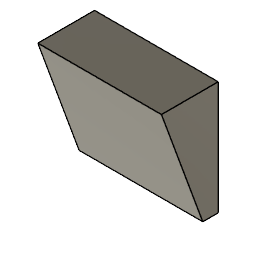
Front Mount (Autodesk Fusion 360 archive; units mm, degrees)
design "Front Bracket"
part number: 2026-01-01-12-06-02-870
Autodesk Fusion 360 part; units mm, degrees
sketch "Sketch1" plane through (0, 0, 0) normal (0, 1, 0) x (1, 0, 0)
  line L0 (0, 0) -> (38, 0)
  line L1 (38, 0) -> (38, -38)
  line L2 (38, -38) -> (0, -38)
  line L3 (0, -38) -> (0, 0)
  circle A0 centre (5, -5) radius 1.35
  circle A1 centre (33, -5) radius 1.35
  circle A2 centre (5, -33) radius 1.35
  circle A3 centre (33, -33) radius 1.35
  line L4 (5, -5) -> (0, -5)
  dimension "d1" = 38
  dimension "d2" = 38
  dimension "d3" = 2.7
  dimension "d4" = 5
  dimension "d5" = 5
  dimension "d6" = 2.7
  dimension "d7" = 2.7
  dimension "d8" = 2.7
  dimension "d9" = 5
  dimension "d10" = 5
  dimension "d11" = 5
  dimension "d12" = 5
  dimension "d13" = 5
  dimension "d14" = 5
  constraint horizontal L0
  constraint vertical L1
  constraint horizontal L2
  constraint vertical L3
  constraint coincident L0.start L3.end
  constraint coincident A0.centre L4.start
  constraint coincident L3 L4.end
  constraint perpendicular L3 L4
  measures "d1" distance of L0.start L0.end
  measures "d2" distance of L0.start L2.end
  measures "d3" diameter of A0
  measures "d4" distance of L3 A0.centre
  measures "d5" distance of L0 A0.centre
  measures "d6" diameter of A1
  measures "d7" diameter of A2
  measures "d8" diameter of A3
  measures "d9" distance of L0 A1.centre
  measures "d10" distance of L1 A1.centre
  measures "d11" distance of L2 A3.centre
  measures "d12" distance of L1 A3.centre
  measures "d13" distance of L3 A2.centre
  measures "d14" distance of L2 A2.centre
ref_plane "WorkPlane1" through (19, 0, 38) normal (0, 0, 1) x (-1, 0, 0)
sketch "Sketch5" plane through (0, 0, 0) normal (1, 0, 0) x (0, 1, 0)
  line L0 (0, 0) -> (48.3488, 0) construction
  line L1 (0, 38) -> (-19.011, 38)
  line L2 (0, 38) -> (0, 0)
  line L3 (-7, 5) -> (-5.1801, 0)
  line L4 (-5.1801, 0) -> (0, 0)
  line L5 (-7, 5) -> (-19.011, 38)
  constraint horizontal L0
  constraint coincident L0.start L2.end
  constraint horizontal L1
  constraint perpendicular L0 L2
  constraint perpendicular L2 L4
  constraint coincident L1 L5.end
  constraint parallel L3 L5
extrude "Extrude2" add sketch "Sketch5" along normal blind 38
extrude "Extrude3" cut sketch "Sketch1" against normal blind 3 contours A0 | A1 | A2 | A3
extrude "Extrude4" add sketch "Sketch5" against normal blind 1.7
extrude "Extrude5" add 1 faces at (38, -8.0637, 25.3333) along direction (1, 0, 0) blind 1.7

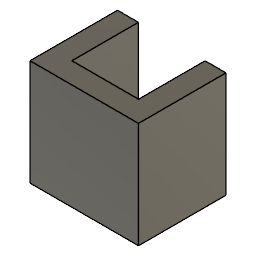
design "Clamp"
part number: 2026-01-01-13-21-08-944
Autodesk Fusion 360 part; units mm, degrees
sketch "Sketch1" plane through (0, 0, 0) normal (0, 0, 1) x (1, 0, 0)
  line L0 (0, 0) -> (0, 25.4)
  line L1 (0, 0) -> (25.4, 0)
  line L2 (25.4, 0) -> (25.4, 25.4)
  line L3 (0, 25.4) -> (-8, 25.4)
  line L4 (-8, -8) -> (33.4, -8)
  line L5 (25.4, 25.4) -> (33.4, 25.4)
  line L6 (-8, 25.4) -> (-8, -8)
  line L7 (33.4, 25.4) -> (33.4, -8)
  dimension "d1" = 25.4
  dimension "d2" = 25.4
  dimension "d3" = 25.4
  dimension "d4" = 8
  dimension "d5" = 8
  dimension "d6" = 8
  constraint coincident L0.start L1.start
  constraint vertical L0
  constraint perpendicular L0 L1
  constraint perpendicular L1 L2
  constraint perpendicular L0 L3
  constraint perpendicular L0 L4
  constraint perpendicular L2 L5
  constraint perpendicular L4 L6
  constraint perpendicular L4 L7
  measures "d1" distance of L0.start L0.end
  measures "d2" distance of L0.start L1.end
  measures "d3" distance of L1.end L2.end
  measures "d4" distance of L0.end L3.end
  measures "d5" distance of L2.end L5.end
  measures "d6" distance of L1 L4
extrude "Extrude1" add sketch "Sketch1" along normal blind 40.439

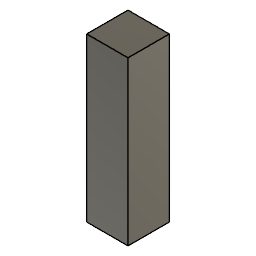
design "Golf Cart Bar"
part number: 2026-01-01-12-43-56-600
Autodesk Fusion 360 part; units mm, degrees
sketch "Sketch2" plane through (0, 0, 0) normal (0, 0, 1) x (1, 0, 0)
  line L0 (0, 0) -> (25.4, 0)
  line L1 (25.4, 0) -> (25.4, 25.4)
  line L2 (25.4, 25.4) -> (0, 25.4)
  line L3 (0, 25.4) -> (0, 0)
  dimension "d4" = 25.4
  dimension "d5" = 25.4
  constraint horizontal L0
  constraint vertical L1
  constraint horizontal L2
  constraint vertical L3
  constraint coincident L0.start L3.end
  measures "d4" distance of L0.start L0.end
  measures "d5" distance of L0.start L2.end
extrude "Extrude1" add sketch "Sketch2" along normal blind 100
